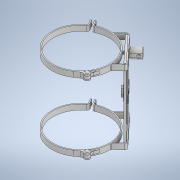
# Autodesk Inventor part: telescope_mount
Saved by Autodesk Inventor 2021.4 (Build 254397000, 397)
## iProperties
Created: 2023-11-22
Part Number: telescope_mount
Material: Generic
Document SubType Name: Modeling
Designer: ZenBook
Density: 1 g/cm^3
Appearance: Default
Author: ZenBook
Autodesk Inventor part; units mm, degrees
ref_plane "YZ Plane" through (0, 0, 0) normal (1, 0, 0) x (0, 1, 0)
ref_plane "XZ Plane" through (0, 0, 0) normal (0, 1, 0) x (-1, 0, 0)
ref_plane "XY Plane" through (0, 0, 0) normal (0, 0, 1) x (1, 0, 0)
derived "skeleton_1.ipt"
sketch "Sketch1" plane through (0, 0, 0) normal (0, 1, 0) x (-1, 0, 0)
  line L0 (0, 0) -> (0, 550)
  circle A0 centre (0, 550) radius 6
  line L1 (0, 550) -> (43.8812, 590.9199)
  line L2 (-15.7936, 654.9134) -> (83.0961, 548.8671)
  line L3 (111.4949, 533.0759) -> (80.291, 566.538)
  line L4 (96.8679, 519.4359) -> (65.6639, 552.898)
  line L5 (0, 0) -> (-350, 0)
  line L6 (11.0017, 632.044) -> (5.1509, 626.588)
  point P0 (0, 440)
sketch "Sketch2" plane through (15.7936, 0, 654.9134) normal (-0.6819984, 0, -0.7313537) x (0, -1, 0)
  line L0 (0, -60) -> (0, 0) construction
  line L1 (0, -72) -> (0, 80)
  circle A0 centre (0, 0) radius 10
  line L2 (10, -4.956) -> (10, -4.9245)
  line L3 (-10, 4.9268) -> (-10, 4.959)
  line L4 (-5, 73) -> (5, 73)
  point P0 (0, 0)
  point P1 (0, 0)
  point P2 (0, 0)
  point P3 (0, 10)
  point P4 (0, 10)
  point P5 (0, 10)
  point P6 (0, -57)
  point P7 (0, 45)
sketch "Sketch3" plane through (-42.7147, 0, 709.4732) normal (-0.7313537, 0, 0.6819984) x (0, -1, 0)
  line L0 (0, 0) -> (0, -145) construction
  line L1 (105, 0) -> (-105, 0)
  circle A0 centre (0, 0) radius 6
  line L2 (0, 50) -> (0, -50)
  line L3 (-105, -80) -> (-105, 80)
  point P0 (0, 0)
  point P1 (0, 0)
  point P2 (0, 0)
  point P3 (0, 0)
  point P4 (-79, -23)
sketch "Sketch4" plane through (15.7936, 0, 654.9134) normal (0.6333709, 0.5, -0.5906279) x (-0.6819984, 0, -0.7313537)
  line L0 (0, 0) -> (145, 0) construction
  line L1 (45, 0) -> (45, -99)
  line L2 (45, -99) -> (39, -99)
sketch "Sketch6" plane through (25.3977, -85.7365, 592.6316) normal (0.7285714, -0.0871445, -0.6794038) x (-0.6819984, 0, -0.7313537)
  line L0 (6, 0) -> (0, 0) construction
  line L1 (0, 0) -> (0, 86.0639)
  line L2 (0, 86.0639) -> (-39, 86.0639)
  point P0 (-5, 86.0639)
  point P1 (4, 0)
  point P2 (-4, 0)
  point P3 (5, 86.0639)
sketch "Sketch8" plane through (68.4511, 0, 605.8095) normal (0.5586604, -0.5735764, 0.5990899) x (-0.7313537, 0, 0.6819984)
  line L0 (0, 0) -> (152, 0) construction
  line L1 (117, 0) -> (117, -111)
  line L2 (117, -111) -> (132, -111)
sketch "Sketch7" plane through (-58.4006, 79, 692.6521) normal (-0.0929708, 0.9906647, -0.099699) x (0.8216319, 0.1328926, 0.554311)
  line L0 (89.7407, 0) -> (4.4573, 19.497)
  line L1 (4.4573, 19.497) -> (0, 0)
  line L2 (93.0837, 14.6227) -> (89.7407, 0)
  point P0 (3.5658, 15.5976)
  point P1 (5.3487, 23.3964)
  point P2 (90.855, 4.8742)
  point P3 (88.6264, -4.8742)
ref_plane "Work Plane1" through (15.7936, 0, 654.9134) normal (-0.6819984, 0, -0.7313537) x (0, -1, 0)
ref_plane "Work Plane2" through (-42.7147, 0, 709.4732) normal (-0.7313537, 0, 0.6819984) x (0, -1, 0)
ref_plane "Work Plane3" through (-8.6147, 0, 746.0409) normal (0.7313537, 0, -0.6819984) x (-0.6819984, 0, -0.7313537)
sketch "Sketch10" plane through (-8.6147, 0, 746.0409) normal (0.7313537, 0, -0.6819984) x (-0.6819984, 0, -0.7313537)
  line L0 (50, -105) -> (50, 105) construction
  line L1 (0, 0) -> (100, 0) construction
  line L2 (100, -105) -> (0, -105)
  line L3 (0, -105) -> (0, 105)
  line L4 (0, 105) -> (100, 105)
  line L5 (100, 105) -> (100, -105)
  line L6 (100, -105) -> (0, 105) construction
  line L7 (0, -105) -> (100, 105) construction
  circle A0 centre (50, 0) radius 6 projected
  line L8 (83, 0) -> (65, 70)
  line L9 (65, 70) -> (50, 70)
  line L10 (17, 0) -> (35, 70)
  line L11 (35, 70) -> (50, 70)
  line L12 (83, 0) -> (65, -70)
  line L13 (65, -70) -> (50, -70)
  line L14 (17, 0) -> (35, -70)
  line L15 (35, -70) -> (50, -70)
  circle A1 centre (50, 0) radius 25
  point P0 (539.7445, 0)
  point P1 (73, 79)
  point P2 (50, 0)
  dimension "d1" = 66
  dimension "d2" = 140
  dimension "d3" = 30
  dimension "d82" = 50
  constraints: 28 end point, 5 midpoint, 5 symmetric about line, 3 perpendicular, 2 parallel, 2 point on line, 1 centre point, 1 coincident
  measures "d1" distance of L8.start L10.start
  measures "d2" distance between parallel lines of L13 L9
  measures "d3" distance of L10.end L8.end
  measures "d82" diameter of A1
extrude "Extrusion10" add sketch "Sketch10" against normal blind 1 contours A1
extrude "Extrusion1" add sketch "Sketch10" against normal blind 2 from surface at -1 separate body contours L12 L13 L15 L14 L10 L11 L9 L8 | A1
extrude "Extrusion2" add sketch "Sketch10" against normal blind 5 from surface at -3 separate body contours L2 L3 L4 L5 | L12 L13 L15 L14 L10 L11 L9 L8 | A1
hole "Hole1" at (-58.4006, 79, 692.6521) direction (-0.7313537, 0, 0.6819984) diameter 8 end through all bodies 2 3
ref_plane "Work Plane4" through (-43.7735, 79, 679.0121) normal (0.0929708, -0.9906647, 0.099699) x (-0.7313537, 0, 0.6819984)
sketch "Sketch11" plane through (-43.7735, 79, 679.0121) normal (0.0929708, -0.9906647, 0.099699) x (-0.7313537, 0, 0.6819984)
  line L0 (25.0021, 0.0215) -> (28, -4) construction
  line L1 (34, 0) -> (34, 4)
  line L2 (34, 4) -> (23, 4)
  line L3 (23, 4) -> (23, 10)
  line L4 (23, 10) -> (18, 10)
  line L5 (18, 10) -> (18, 13)
  line L6 (18, 13) -> (-8, 13)
  line L7 (-8, 13) -> (-8, 0)
  line L8 (-8, 0) -> (34, 0)
  line L9 (23, -4) -> (23, 4) projected
  line L10 (0, -87.4837) -> (0, 0) construction
  line L11 (0, 0) -> (20, 0) projected
  point P0 (-495.0991, 473.1567)
  point P1 (0, 13)
  dimension "d17" = 11
  dimension "d18" = 5
  dimension "d19" = 31
  dimension "d21" = 26
  dimension "d22" = 20
  constraints: 18 end point, 7 perpendicular, 3 point on line, 2 collinear
  measures "d17" distance between parallel lines of L1 L3
  measures "d18" distance between parallel lines of L5 L3
  measures "d19" distance between parallel lines of L3 L7
  measures "d21" diameter of L6 L11
  measures "d22" diameter of L4 L11
revolve "Revolution1" add sketch "Sketch11" angle 360 about axis through (-43.7735, 79, 679.0121) along (-0.7313537, 0, 0.6819984) separate body
ref_plane "Work Plane5" through (-52.5568, 77.2278, 669.5933) normal (-0.6756317, -0.1363212, -0.7245263) x (0.1977827, -0.9802459, 0)
sketch "Sketch12" plane through (-52.5568, 77.2278, 669.5933) normal (-0.6756317, -0.1363212, -0.7245263) x (0.1977827, -0.9802459, 0)
  circle A0 centre (0, 0) radius 4
  point P0 (86.0971, -487.7752)
  point P1 (-0.5786, 3.9579)
  constraints: 1 coincident, 3 other
extrude "Extrusion12" cut sketch "Sketch12" against normal through all bodies 4
sketch "Sketch13" plane through (-82.6654, 105, 678.3615) normal (0, 1, 0) x (0.6819984, 0, 0.7313537)
  line L0 (100, 5) -> (0, 5) projected
  line L1 (100, 0) -> (100, 5) projected
  line L2 (0, 5) -> (0, 0) projected
  line L3 (100, 5) -> (0, 5)
  arc A0 (0, 5) -> (-3, 2) centre (0, 2) ccw
  line L4 (-3, 2) -> (-3, -25.43)
  arc A1 (-4.8837, -29.7954) -> (-3, -25.43) centre (-9, -25.43) ccw
  arc A2 (-4.8837, -29.7954) -> (104.8837, -29.7954) centre (50, -88) ccw
  arc A3 (103, -25.43) -> (104.8837, -29.7954) centre (109, -25.43) ccw
  line L5 (103, -25.43) -> (103, 2)
  arc A4 (103, 2) -> (100, 5) centre (100, 2) ccw
  arc A5 (-6.9419, -27.6127) -> (106.9419, -27.6127) centre (50, -88) ccw
  arc A6 (-6.9419, -27.6127) -> (-6, -25.43) centre (-9, -25.43) ccw
  line L6 (-6, -25.43) -> (-6, 2)
  arc A7 (0, 8) -> (-6, 2) centre (0, 2) ccw
  line L7 (0, 8) -> (100, 8)
  arc A8 (106, 2) -> (100, 8) centre (100, 2) ccw
  line L8 (106, 2) -> (106, -25.43)
  arc A9 (106, -25.43) -> (106.9419, -27.6127) centre (109, -25.43) ccw
  arc A10 (104.8837, -29.7954) -> (-4.8837, -29.7954) centre (50, -88) ccw
  line L9 (53.5971, -8) -> (44.2082, -8)
  line L10 (100, 0) -> (0, 0) projected
  line L11 (50, -88) -> (-155.0851, -44.4078) construction
  line L12 (-48.4385, -70.1433) -> (-34.2825, -73.1522)
  arc A11 (-29.5628, -79.6475) -> (-34.2825, -73.1522) centre (-35.53, -79.0211) ccw
  line L13 (-48.4385, -70.1433) -> (-49.0622, -73.0777)
  line L14 (-49.0622, -73.0777) -> (-34.9063, -76.0867)
  arc A12 (-32.5464, -79.3343) -> (-34.9063, -76.0867) centre (-35.53, -79.0211) ccw
  line L15 (-47.191, -64.2744) -> (-33.0351, -67.2833)
  arc A13 (-33.0351, -67.2833) -> (-26.0815, -63.2693) centre (-31.7876, -61.4144) ccw
  line L16 (-47.191, -64.2744) -> (-46.5673, -61.3399)
  line L17 (-46.5673, -61.3399) -> (-32.4113, -64.3489)
  arc A14 (-32.4113, -64.3489) -> (-28.9345, -62.3419) centre (-31.7876, -61.4144) ccw
  line L18 (50, -88) -> (50, 0) construction
  line L19 (0, 0) -> (100, 0) projected
  circle A15 centre (136.1707, -72.8058) radius 7.5
  circle A16 centre (136.1707, -72.8058) radius 3
  line L20 (50, -88) -> (136.1707, -72.8058) construction
  line L21 (122.9728, -48.4529) -> (129.8451, -61.1337)
  arc A17 (129.8451, -61.1337) -> (136.5132, -65.3136) centre (136.8786, -57.322) ccw
  line L22 (136.8786, -57.322) -> (129.8451, -61.1337) construction
  line L23 (136.8786, -57.322) -> (136.5132, -65.3136) construction
  line L24 (132.0979, -100.204) -> (134.2186, -85.9374)
  arc A18 (139.055, -79.729) -> (134.2186, -85.9374) centre (142.1317, -87.1137) ccw
  line L25 (-32.5464, -79.3343) -> (-29.5628, -79.6475)
  line L26 (-28.9345, -62.3419) -> (-26.0815, -63.2693)
  arc A19 (106.9419, -27.6127) -> (-6.9419, -27.6127) centre (50, -88) ccw
  point P0 (-439.7445, 523.0991)
  point P1 (128.7846, -74.1081)
  point P2 (130.5223, -67.8716)
  point P3 (132.5506, -79.3743)
  point P4 (132.0979, -100.204)
  point P5 (139.055, -79.729)
  point P6 (103.0926, -13.8891)
  point P7 (-3.0926, -13.8891)
  point P8 (-3, -24.1251)
  point P9 (103, -24.1251)
  point P10 (-30.3625, -67.2428)
  dimension "d41" = 15
  dimension "d31" = 3
  dimension "d32" = 3
  dimension "d34" = 20
  dimension "d35" = 6
  dimension "d36" = 78
  dimension "d39" = 80
  dimension "d40" = 90
  dimension "d42" = 6
  dimension "d43" = 8
  dimension "d91" = 5
  dimension "d92" = 80
  constraints: 44 end point, 42 point on circle, 19 centre point, 18 tangent, 9 symmetric about line, 6 perpendicular, 5 equal radius, 5 point on line, 3 coincident, 3 concentric, 3 parallel, 1 collinear, 1 horizontal, 1 midpoint, 12 other
  measures "d31" distance between parallel lines of L7 L0
  measures "d32" radius of A0
  measures "d34" distance edge to line of A2 L13
  measures "d35" distance between parallel lines of L15 L12
  measures "d36" angle of L18 L11
  measures "d39" angle of L18 L20
  measures "d40" angle of L21 L22
  measures "d42" diameter of A16
  measures "d43" radius of A17
  measures "d91" distance edge to line of A19 L10
  measures "d92" radius of A2
extrude "Extrusion3" add sketch "Sketch13" against normal blind 15 separate body contours L0 A0 L4 A19 A6 L6 A7 L7 A8 L8 A9 L5 A4 | A19 A5 A15 A2 A3 L5 | L5 A3 A10 A1 L4 A19 | L4 A1 A2 L26 A5 A19 | L26 A13 A5 | A5 A13 L15 L16 L17 A14 | A15 A5 picked at (130.7393, -73.7635)
extrude "Extrusion4" add sketch "Sketch13" against normal blind 15 separate body contours A15 A5 L25 A2 | A15 A5 | L25 A5 A11 | A5 A12 L14 L13 L12 A11 picked at (130.7393, -73.7635)
ref_plane "Work Plane6" through (-82.6654, 97.5, 678.3615) normal (0, 1, 0) x (0.6819984, 0, 0.7313537)
extrude "Extrusion5" add sketch "Sketch13" against normal blind 15 contours A15 A5 | A15 A18 L24 A5 picked at (131.9419, -70.1202) bodies 6
extrude "Extrusion6" cut sketch "Sketch13" against normal mid plane 8 from surface at -7.5 contours L21 A17 A15 A5 | A15 A5 | A15 A5 bodies 6
extrude "Extrusion7" add sketch "Sketch13" along normal mid plane 8 from surface at -7.5 contours L21 A17 A15 A5 | A15 A5 | A15 A5 bodies 5
ref_plane "Work Plane7" through (-43.044, 105, 827.6039) normal (0.7986355, 0, 0.601815) x (0, 1, 0)
sketch "Sketch14" plane through (-43.044, 105, 827.6039) normal (0.7986355, 0, 0.601815) x (0, 1, 0)
  line L0 (0, 3) -> (0, -3) construction
  line L1 (-3.5, 3) -> (0, 3) construction
  line L2 (-15, -3) -> (-15, 3) construction
  line L3 (-15, 4.5) -> (-15, 3)
  line L4 (-15, 3) -> (0, 3)
  line L5 (0, 3) -> (0, 4.5)
  arc A0 (0, -4.5) -> (0, 4.5) centre (0, 0) ccw
  line L6 (0, -4.5) -> (0, -3)
  line L7 (0, -3) -> (-15, -3)
  line L8 (-15, -3) -> (-15, -4.5)
  arc A1 (-15, 4.5) -> (-15, -4.5) centre (-15, 0) ccw
  line L9 (-15, 0) -> (0, 0)
  line L10 (-19.5, 0) -> (4.5, 0)
  line L11 (-3.5, 0) -> (-11.5, 0) projected
  point P0 (-105, -686.8584)
  point P1 (0, 0)
  dimension "d54" = 4.5
  constraints: 16 end point, 6 collinear, 6 point on circle, 4 symmetric about line, 3 perpendicular, 3 point on line, 2 centre point, 2 midpoint, 1 equal radius
  measures "d54" radius of A0
revolve "Revolution2" add sketch "Sketch14" angle 360 about axis through (-43.044, 85.5, 827.6039) along (0, 1, 0) separate body contours L10 L9 A0 L6 L7 L8 A1
sketch "Sketch15" plane through (-162.1177, 105, 704.7237) normal (-0.8571673, 0, 0.5150381) x (0, 1, 0)
  line L0 (-15, -2.9835) -> (-15, 0) construction
  line L1 (0, 0) -> (0, 14.4722) construction
  line L2 (-15, 0) -> (0, 14.4722) construction
  line L3 (0, 0) -> (-15, 0) construction
  line L4 (0, 14.4722) -> (-15, 14.4722) construction
  line L5 (0, 0) -> (-15, 14.4722) construction
  point P0 (-105, 520.5693)
  point P1 (-7.5, 7.2361)
  constraints: 4 end point, 1 midpoint
hole "Hole3" at (-165.8446, 97.5, 698.5211) direction (0.8571673, 0, -0.5150381) diameter 8 end through all bodies 6 5
ref_plane "Work Plane8" through (-82.6654, 0, 678.3615) normal (0, 1, 0) x (0.6819984, 0, 0.7313537)
mirror "Mirror1" about plane through (-82.6654, 0, 678.3615) normal (0, 1, 0) bodies 6 5 7
sketch "Sketch16" plane through (-76.8146, 105, 672.9055) normal (0.7313537, 0, -0.6819984) x (0, 1, 0)
  line L0 (0, 100) -> (-15, 100) construction
  line L1 (0, 0) -> (-15, 0) construction
  line L2 (-7.5, 0) -> (-7.5, 100) construction
  point P0 (-105, -439.7445)
  point P1 (-7.5, 77.5188)
  point P2 (-7.5, 22.4812)
  dimension "d63" = 22.4812
  dimension "d64" = 22.4812
  constraints: 2 end point, 2 midpoint, 2 point on line, 1 perpendicular
  measures "d63" distance from line of L0 point (-7.5, 77.519)
  measures "d64" distance from line of L1 point (-7.5, 22.481)
hole "Hole4" at (-23.9469, 97.5, 729.5992) at (-61.4824, 97.5, 689.3472) direction (-0.7313537, 0, 0.6819984) diameter 6 depth 8 tip angle 118 bodies 5 3
mirror "Mirror3" about plane through (-82.6654, 0, 678.3615) normal (0, 1, 0) of "Hole4" bodies 5 3
thread "Thread1" size "M8x1.25" class "6g" standard "ISO Metric profile" full length
sketch "Sketch17" plane through (-14.4656, -105, 751.4969) normal (-0.7313537, 0, 0.6819984) x (0, 1, 0)
  circle A0 centre (105, 50) radius 6 projected
  circle A1 centre (105, 50) radius 20
  line L0 (115.5, 56.0622) -> (115.5, 43.9378)
  line L1 (115.5, 43.9378) -> (105, 37.8756)
  line L2 (105, 37.8756) -> (94.5, 43.9378)
  line L3 (94.5, 43.9378) -> (94.5, 56.0622)
  line L4 (94.5, 56.0622) -> (105, 62.1244)
  line L5 (105, 62.1244) -> (115.5, 56.0622)
  line L6 (105, 0) -> (105, 100) construction
  dimension "d74" = 40
  dimension "d75" = 21
  constraints: 12 end point, 2 coincident, 1 centre point, 1 point on line, 13 other
  measures "d74" diameter of A1
  measures "d75" distance between parallel lines of L1 L4
extrude "Extrusion8" add sketch "Sketch17" along normal blind 2 separate body contours A1 | L0 L1 L2 L3 L4 L5
extrude "Extrusion9" add sketch "Sketch17" along normal blind 5 from surface at 2 contours L0 L1 L2 L3 L4 L5 bodies 8
thread "Thread2" size "M12x1.75" class "6H" standard "ISO Metric profile" full length
ref_plane "Work Plane9" through (-43.7735, 79, 679.0121) normal (0.0929708, -0.9906647, 0.099699) x (-0.7313537, 0, 0.6819984)
sketch "Sketch18" plane through (-43.7735, 79, 679.0121) normal (0.0929708, -0.9906647, 0.099699) x (-0.7313537, 0, 0.6819984)
  line L0 (-8, -13) -> (18, -13) projected
  line L1 (-8, 13) -> (18, 13) projected
  line L2 (18, -13) -> (18, -12)
  line L3 (18, -12) -> (-8, -12)
  line L4 (-8, -12) -> (-8, -13)
  line L5 (-8, 13) -> (-8, 12)
  line L6 (-8, 12) -> (18, 12)
  line L7 (18, 12) -> (18, 13)
  point P0 (-495.0991, 473.1567)
  dimension "d85" = 1
  dimension "d86" = 1
  constraints: 12 end point, 6 perpendicular
  measures "d85" distance between parallel lines of L0 L3
  measures "d86" distance between parallel lines of L1 L6
extrude "Extrusion11" cut sketch "Sketch18" against normal through all both and the other way through all bodies 4
equation "\"d32\" = d31"
equation "\"d64\" = d63"
